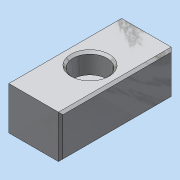
# Autodesk Inventor part: BC-10025
Saved by Autodesk Inventor 2016 (Build 200138000, 138)
## iProperties
Created: 2015-12-03
Part Number: BC-10025
Project: DIPOLO BC-3T- SIRIUS
Cost Center: 1504002005
Material: Aço Inox AISI 304
Document SubType Name: Modeling
Designer: reinaldo.basilio
Density: 8 g/cm^3
Appearance: Chrome - Satin
Description: Chaveta de posicionamento transversal das partes inferior e superior.
Mass: 20.4954 g
Surface Area: 13.9947 cm^2
Volume: 2.56193 cm^3
RuleStatus: InUse
AfterMaterialChange0: file://_iMaterial
AfterAnyiPropertyChange0: file://_iMaterial
AfterDocNew0: file://_Naming_par
AfterDocNew1: file://_NameStart
AfterDocNew2: file://_NameStart1
AfterDocNew3: file://_Materiais
DocNumber: XXXXX-XXX-XXXX-00-001.ipt
Folder: .
Title: DIPOLO BC-3T- SIRIUS
Author: reinaldo.basilio
Subject: BC-10025
Autodesk Inventor part; units mm, degrees
ref_plane "YZ Plane" through (0, 0, 0) normal (1, 0, 0) x (0, 1, 0)
ref_plane "XZ Plane" through (0, 0, 0) normal (0, 1, 0) x (-1, 0, 0)
ref_plane "XY Plane" through (0, 0, 0) normal (0, 0, 1) x (1, 0, 0)
sketch "Sketch5" plane through (0, 0, 0) normal (0, 0, 1) x (1, 0, 0)
  line L0 (-12.5, 6) -> (12.5, 6)
  line L1 (12.5, 6) -> (12.5, -6)
  line L2 (12.5, -6) -> (-12.5, -6)
  line L3 (-12.5, -6) -> (-12.5, 6)
  point P0 (0, 0)
  point P1 (0, 6)
  point P2 (12.5, 0)
  dimension "d8" = 25
  dimension "d9" = 12
  constraints: 8 end point, 2 midpoint, 2 parallel, 1 horizontal, 1 horizontal alignment, 1 perpendicular, 1 vertical alignment
  measures "d8" distance of L0.start L0.end
  measures "d9" distance of L2.end L0.start
extrude "Extrusion5" add sketch "Sketch5" along normal blind 9.5
sketch "Sketch6" plane through (0, 0, 9.5) normal (0, 0, 1) x (1, 0, 0)
  circle A0 centre (0, 0) radius 2
  dimension "d12" = 4
  constraints: 1 centre point, 1 coincident
  measures "d12" diameter of A0
hole "Hole1" at (0, 0, 9.5) direction (0, 0, -1) diameter 4.2 end through all counterbore diameter 7.5 counterbore depth 4.5 clearance for "Socket Head Cap Screw DIN EN ISO 4762" size "M4" standard "DIN"
chamfer "Chamfer2" distance 0.5 angle 45 4 edges at (0, -6, 9.5) (0, 6, 9.5) (0, -6, 0) (0, 6, 0)
chamfer "Chamfer3" distance 0.5 angle 45 4 edges at (12.5, 6, 4.75) (-12.5, 6, 4.75) (-12.5, -6, 4.75) (12.5, -6, 4.75)
chamfer "Chamfer4" distance 0.5 angle 45 1 edges at (0, 3.75, 9.5)
body "Solid5"
